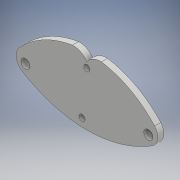
# Autodesk Inventor part: nariz
Saved by Autodesk Inventor 2018 (Build 220112000, 112)
## iProperties
Created: 2019-01-30
Part Number: nariz
Material: Generic
Document SubType Name: Modeling
Designer: Estudiante
Density: 1 g/cm^3
Appearance: Default
Author: Estudiante
Autodesk Inventor part; units mm, degrees
ref_plane "YZ Plane" through (0, 0, 0) normal (1, 0, 0) x (0, 1, 0)
ref_plane "XZ Plane" through (0, 0, 0) normal (0, 1, 0) x (-1, 0, 0)
ref_plane "XY Plane" through (0, 0, 0) normal (0, 0, 1) x (1, 0, 0)
sketch "Sketch1" plane through (0, 0, 0) normal (0, 1, 0) x (-1, 0, 0)
  arc A0 (-25, 0) -> (0, 0) centre (-12.5, 15.6125) ccw
  arc A1 (0, 0) -> (-25, 0) centre (-12.5, -8.2916) ccw
  dimension "d0" = 25
  dimension "d1" = 20
  dimension "d2" = 15
  constraints: 4 point on circle, 2 centre point
  measures "d0" distance of A0.end A0.start
  measures "d1" radius of A0
  measures "d2" radius of A1
extrude "Extrusion1" add sketch "Sketch1" along normal blind 1
fillet "Fillet1" radius 2 2 edges at (25, 0.5, 0) (0, 0.5, 0)
sketch "Sketch2" plane through (0, 1, 0) normal (0, 1, 0) x (1, 0, 0)
  arc A0 (1.3645, -1.7583) -> (23.6355, -1.7583) centre (12.5, 8.2916) ccw projected
  arc A1 (1.3645, -1.7583) -> (23.6355, -1.7583) centre (12.5, 8.2916) ccw projected
  arc A2 (9.4548, -6.3961) -> (12.5, -5.3578) centre (10.2741, -3.8143) ccw
  arc A3 (12.5, -5.3578) -> (15.5452, -6.3961) centre (14.7259, -3.8143) ccw
  line L0 (9.4548, -6.3961) -> (10.705, -7.1711)
  line L1 (10.705, -7.1711) -> (14.8328, -7.2667)
  line L2 (14.8328, -7.2667) -> (15.5452, -6.3961)
  point P0 (0, 0)
  constraints: 6 end point, 5 point on circle, 2 centre point
extrude "Extrusion2" cut sketch "Sketch2" against normal blind 1 contours A2 A0 A3 L2 L1 L0 | A2 A3 A0
sketch "Sketch3" plane through (0, 1, 0) normal (0, 1, 0) x (1, 0, 0)
  arc A0 (1.7769, 1.2699) -> (1.3645, -1.7583) centre (2.8492, -0.4183) ccw projected
  line L0 (0.8935, 0) -> (2.3935, 0)
  arc A1 (23.6355, -1.7583) -> (23.2231, 1.2699) centre (22.1508, -0.4183) ccw projected
  line L1 (24.1065, 0) -> (22.6065, 0)
  circle A2 centre (2.3935, 0) radius 0.75
  circle A3 centre (22.6065, 0) radius 0.75
  circle A4 centre (11.6968, 3.0289) radius 0.5
  point P0 (0, 0)
  dimension "d10" = 1.5
  dimension "d11" = 1.5
  dimension "d12" = 1.5
  dimension "d13" = 1.5
  dimension "d14" = 1
  constraints: 4 end point, 3 centre point, 2 coincident, 2 horizontal, 2 point on circle
  measures "d10" distance of L0.start L0.end
  measures "d11" distance of L1.start L1.end
  measures "d12" diameter of A2
  measures "d13" diameter of A3
  measures "d14" diameter of A4
extrude "Extrusion3" cut sketch "Sketch3" against normal blind 1
sketch "Sketch4" plane through (0, 1, 0) normal (0, 1, 0) x (1, 0, 0)
  circle A0 centre (12.5028, -4.4622) radius 0.5
  point P0 (0, 0)
  dimension "d17" = 1
  constraints: 1 centre point
  measures "d17" diameter of A0
extrude "Extrusion4" cut sketch "Sketch4" against normal blind 1
body "Solid1"
